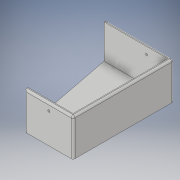
# Autodesk Inventor part: Dumping bin
Saved by Autodesk Inventor 2019 (Build 230136000, 136)
## iProperties
Created: 2019-01-04
Part Number: Dumping bin
Material: Generic
Document SubType Name: Modeling
Designer: scdrobotics
Density: 1 g/cm^3
Appearance: Default
Author: scdrobotics
## iProperties of the stored document Dumping bin_3DPrint.ipt
Created: 2019-01-04
Part Number: Dumping bin_3DPrint
Material: Generic
Document SubType Name: Modeling
Designer: scdrobotics
Density: 1 g/cm^3
Appearance: Default
Author: scdrobotics
Autodesk Inventor part; units mm, degrees
ref_plane "YZ Plane" through (0, 0, 0) normal (1, 0, 0) x (0, 1, 0)
ref_plane "XZ Plane" through (0, 0, 0) normal (0, 1, 0) x (-1, 0, 0)
ref_plane "XY Plane" through (0, 0, 0) normal (0, 0, 1) x (1, 0, 0)
sketch "Sketch1" plane through (0, 0, 0) normal (0, 1, 0) x (-1, 0, 0)
  line L0 (0, 0) -> (82.55, 0)
  line L1 (114.3, -165.1) -> (0, -165.1)
  line L2 (0, -165.1) -> (0, 0)
  line L3 (82.55, 0) -> (114.3, -88.9)
  line L4 (114.3, -88.9) -> (114.3, -165.1)
  line L5 (4.7625, -160.3375) -> (109.5375, -160.3375)
  line L6 (109.5375, -160.3375) -> (109.5375, -89.7249)
  line L7 (109.5375, -89.7249) -> (79.1938, -4.7625)
  line L8 (79.1938, -4.7625) -> (4.7625, -4.7625)
  line L9 (4.7625, -4.7625) -> (4.7625, -160.3375)
  line L10 (109.5375, -160.3375) -> (109.5375, -165.1)
  line L11 (79.1938, -4.7625) -> (79.1938, 0)
  dimension "d0" = 114.3
  dimension "d2" = 4.7625
  constraints: 24 end point, 2 parallel, 2 perpendicular, 2 point on line, 1 horizontal, 1 vertical, 4 other
  measures "d0" distance of L1.start L1.end
  measures "d2" distance between parallel lines of L1 L5
extrude "Extrusion1" add sketch "Sketch1" along normal blind 60.96 contours L0 L11 L8 L9 L5 L10 L1 L2
sketch "Sketch2" plane through (0, 0, 0) normal (0, -1, 0) x (1, 0, 0)
  line L0 (-4.7625, -160.3375) -> (-4.7625, -4.7625) projected
  line L1 (-109.5375, -160.3375) -> (-4.7625, -160.3375) projected
  line L2 (-4.7625, -4.7625) -> (-79.375, -4.7625)
  line L3 (-109.5375, -160.3375) -> (-4.7625, -160.3375)
  line L4 (-4.7625, -160.3375) -> (-4.7625, -4.7625)
  line L5 (-79.375, -4.7625) -> (-109.5375, -160.3375)
  point P0 (0, 0)
  constraints: 8 end point, 1 horizontal, 1 parallel
extrude "Extrusion2" add sketch "Sketch2" against normal blind 5.08
fillet "Fillet1" radius 3.175 1 edges at (-79.375, 2.54, -4.7625)
sketch "Sketch3" plane through (-79.1938, 0, 0) normal (0, 0, 1) x (1, 0, 0)
  line L0 (0, 0) -> (79.1938, 0) projected
  line L1 (-30.3437, 60.96) -> (74.4313, 60.96) projected
  circle A0 centre (39.5969, 49.53) radius 1.651
  dimension "d9" = 3.302
  constraints: 1 centre point
  measures "d9" diameter of A0
hole "Hole1" at (-39.5969, 49.53, 0) direction (0, 0, -1) diameter 3.302 end through all
fillet "Fillet2" radius 3.175 7 edges at (-39.5969, 60.96, 0) (0, 30.48, 0) (-79.1938, 30.48, 0) (0, 60.96, -82.55) (0, 30.48, -165.1) (-54.7688, 60.96, -165.1) (-109.5375, 30.48, -165.1)
body "Solid1"
